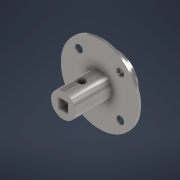
# Autodesk Inventor part: tuk-tukan
Saved by Autodesk Inventor 2021.3 (Build 253353000, 353)
## iProperties
Created: 2021-10-18
Part Number: tuk-tukan
Material: Stainless Steel
Document SubType Name: Modeling
Designer: ASUS
Density: 8 g/cm^3
Appearance: Semi-Polished
Author: ASUS
Autodesk Inventor part; units mm, degrees
ref_plane "YZ Plane" through (0, 0, 0) normal (1, 0, 0) x (0, 1, 0)
ref_plane "XY Plane" through (0, 0, 0) normal (0, 0, 1) x (1, 0, 0)
sketch "Sketch1" plane through (0, 0, 0) normal (0, 0, 1) x (1, 0, 0)
  circle A0 centre (0, 0) radius 16
  line L0 (0, 0) -> (0, 8.955)
  circle A1 centre (0, 0) radius 8.955
  dimension "d0" = 32
  dimension "d1" = 8.955
  constraints: 2 coincident, 2 end point, 1 centre point, 1 vertical, 1 vertical alignment, 2 other
  measures "d0" diameter of A0
  measures "d1" distance of L0.start L0.end
extrude "Extrusion1" add sketch "Sketch1" against normal blind 1 contours A0 | A1
extrude "Extrusion2" add sketch "Sketch1" against normal blind 7 contours A1
sketch "Sketch2" plane through (0, 0, -7) normal (0, 0, -1) x (-1, 0, 0)
  circle A0 centre (0, 0) radius 8.455
  dimension "d6" = 16.91
  constraints: 1 centre point, 1 coincident
  measures "d6" diameter of A0
extrude "Extrusion3" cut sketch "Sketch2" against normal blind 5
sketch "Sketch3" plane through (0, 0, 0) normal (0, 0, 1) x (1, 0, 0)
  circle A0 centre (0, 0) radius 5
  dimension "d9" = 10
  constraints: 1 centre point, 1 coincident
  measures "d9" diameter of A0
extrude "Extrusion4" add sketch "Sketch3" along normal blind 15
sketch "Sketch4" plane through (0, 0, 15) normal (0, 0, 1) x (1, 0, 0)
  line L0 (-2, 2) -> (2, 2)
  line L1 (2, 2) -> (2, -2)
  line L2 (2, -2) -> (-2, -2)
  line L3 (-2, -2) -> (-2, 2)
  line L4 (-2, 2) -> (2, -2) construction
  line L5 (2, 2) -> (-2, -2) construction
  point P0 (0, 0)
  dimension "d12" = 4
  dimension "d13" = 4
  constraints: 12 end point, 2 midpoint, 2 parallel, 1 horizontal, 1 perpendicular
  measures "d12" distance of L1.end L2.end
  measures "d13" distance of L0.end L1.end
extrude "Extrusion5" cut sketch "Sketch4" against normal through all
ref_plane "Work Plane1" through (0, 5.25, 0) normal (0, 1, 0) x (-1, 0, 0)
sketch "Sketch5" plane through (0, 5.25, 0) normal (0, 1, 0) x (-1, 0, 0)
  circle A0 centre (0, 7.5) radius 1.5
  point P0 (0, 0)
  dimension "d17" = 3
  constraints: 1 centre point
  measures "d17" diameter of A0
extrude "Extrusion6" cut sketch "Sketch5" against normal through all
thread "Thread1" size "M3x0.5" class "6H" standard "ANSI Metric M Profile" full length
thread "Thread2" size "M3x0.5" class "6H" standard "ANSI Metric M Profile" full length
sketch "Sketch7" plane through (0, 0, -1) normal (0, 0, -1) x (-1, 0, 0)
  circle A0 centre (0, 0) radius 5 projected
  line L0 (0, 0) -> (8.4853, 8.4853)
  line L1 (0, 0) -> (12, 0) construction
  circle A1 centre (8.4853, 8.4853) radius 1.5
  dimension "d24" = 12
  dimension "d25" = 45
  dimension "d26" = 3
  constraints: 4 end point, 1 centre point, 1 coincident, 1 equal length, 1 horizontal
  measures "d24" distance of L0.start L0.end
  measures "d25" angle of L1 L0
  measures "d26" diameter of A1
extrude "Extrusion7" cut sketch "Sketch7" against normal through all contours A1
thread "Thread3" size "M3x0.5" class "6H" standard "ANSI Metric M Profile" full length
pattern_circular "Circular Pattern1" count 4 over 360 about axis through (0, 0, 0) along (0, 0, -1) of "Extrusion7"
thread "Thread4" size "M3x0.5" class "6H" standard "ANSI Metric M Profile" full length
thread "Thread5" size "M3x0.5" class "6H" standard "ANSI Metric M Profile" full length
thread "Thread6" size "M3x0.5" class "6H" standard "ANSI Metric M Profile" full length
body "Solid1"
